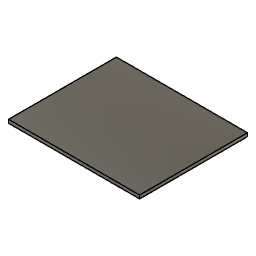
bdn9-smaller-plate (Autodesk Fusion 360 design; units mm, degrees)
Autodesk Fusion 360 part; units mm, degrees
sketch "Sketch1" plane through (0, 0, 0) normal (0, 0, 1) x (1, 0, 0)
  line L0 (0, 0) -> (-79, 0)
  line L1 (-79, 0) -> (-79, -65)
  line L2 (-79, -65) -> (0, -65)
  line L3 (0, -65) -> (0, 0)
  dimension "d1" = 79
  dimension "d2" = 65
  constraint horizontal L0
  constraint vertical L1
  constraint horizontal L2
  constraint vertical L3
  constraint coincident L0.start L3.end
  measures "d1" distance of L0.start L0.end
  measures "d2" distance of L0.start L2.end
extrude "Extrude1" add sketch "Sketch1" along normal blind 2
